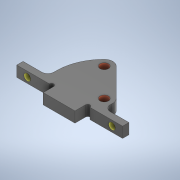
# Autodesk Inventor part: Camera_side_frame
Saved by Autodesk Inventor 2020 (Build 240168000, 168)
## iProperties
Part Number: Camera_side_frame
Material: アセタール樹脂、黒
Document SubType Name: Modeling
Designer: Masato Kubotera
Density: 1.425 g/cm^3
Appearance: 滑らか - 黒
Mass: 4.22239 g
Surface Area: 20.7437 cm^2
Volume: 2.96308 cm^3
Description: POM T5
Author: Masato Kubotera
Autodesk Inventor part; units mm, degrees
ref_plane "YZ Plane" through (0, 0, 0) normal (1, 0, 0) x (0, 1, 0)
ref_plane "XZ Plane" through (0, 0, 0) normal (0, 1, 0) x (-1, 0, 0)
ref_plane "XY Plane" through (0, 0, 0) normal (0, 0, 1) x (1, 0, 0)
derived "Head_basis.ipt"
sketch "スケッチ1" plane through (0, 0, 0) normal (0, 1, 0) x (-1, 0, 0)
  line L0 (-42.9267, 78.5217) -> (-71.5015, 49.9469) construction
  line L1 (6.295, 37.8) -> (-10.705, 37.8) construction
  line L2 (-2.205, 37.8) -> (-42.9267, 78.5217) construction
  line L3 (-2.205, 37.8) -> (-2.205, 4.9887) construction
  line L4 (-54.8845, 55.9573) -> (-58.42, 59.4928) construction
  line L5 (-58.42, 59.4928) -> (-81.0474, 36.8654) construction
  line L6 (-81.0474, 36.8654) -> (-77.5119, 33.3299) construction
  line L7 (-77.5119, 33.3299) -> (-54.8845, 55.9573) construction
  line L8 (-54.8845, 55.9573) -> (-81.0474, 36.8654) construction
  line L9 (-58.42, 59.4928) -> (-77.5119, 33.3299) construction
  line L10 (-60.2972, 54.08) -> (-70.9038, 43.4734) construction
  circle A0 centre (-60.1878, 54.1895) radius 1.6 construction
  line L11 (-56.6522, 57.725) -> (-79.2796, 35.0976) construction
  line L12 (3.8601, -2.5) -> (3.8601, 2.5) construction
  line L13 (5.295, -2.5) -> (5.295, 2.5)
  line L14 (10.8483, 2.5) -> (7.6861, 2.5) construction
  line L15 (-9.705, -2.5) -> (-9.705, 2.5)
  line L16 (5.6869, 2.5) -> (7.6861, 2.5) construction
  arc A1 (5.295, -2.5) -> (7.395, -2.5) centre (6.345, -2.5) ccw
  line L17 (9.935, -2.5) -> (11.935, -2.5) construction
  line L18 (7.395, -2.5) -> (22.795, -2.5)
  line L19 (22.795, -2.5) -> (22.795, -5.5)
  line L20 (22.795, -5.5) -> (14.045, -5.5)
  line L21 (17.795, -2.5) -> (17.795, -5.5) construction
  arc A2 (-11.805, -2.5) -> (-9.705, -2.5) centre (-10.755, -2.5) ccw
  line L22 (-11.805, -2.5) -> (-27.205, -2.5)
  line L23 (-27.205, -2.5) -> (-27.205, -5.5)
  line L24 (-22.205, -2.5) -> (-22.205, -5.5) construction
  line L25 (-18.455, -5.5) -> (-27.205, -5.5)
  circle A3 centre (-11.5577, -9.5) radius 2
  arc A4 (14.045, -5.5) -> (11.1091, -8.5601) centre (14.045, -8.4384) ccw
  line L26 (15.045, -5.5) -> (15.045, -6.9) construction
  line L27 (15.045, -6.9) -> (20.545, -6.9) construction
  line L28 (20.545, -5.5) -> (20.545, -6.9) construction
  circle A5 centre (-11.5577, -9.5) radius 4
  line L29 (22.795, -2.5) -> (22.795, 0.5)
  line L30 (-2.205, -12.0113) -> (-2.205, 4.9887) construction
  line L31 (-19.455, -5.5) -> (-19.455, -6.9) construction
  line L32 (-19.455, -6.9) -> (-24.955, -6.9) construction
  line L33 (-24.955, -5.5) -> (-24.955, -6.9) construction
  line L34 (-69.7337, 48.1791) -> (-66.1982, 44.6436) construction
  circle A6 centre (-75.7441, 38.6332) radius 1.6
  circle A7 centre (1.6555, -22.7132) radius 2
  arc A8 (4.4839, -25.5416) -> (11.1091, -8.5601) centre (-11.5577, -9.5) ccw
  line L35 (-14.3861, -12.3284) -> (-1.1729, -25.5416)
  circle A9 centre (1.6555, -22.7132) radius 4
  line L36 (4.4839, -19.8848) -> (-8.7293, -6.6716)
  line L37 (1.6555, -22.7132) -> (-11.5577, -9.5) construction
  line L38 (-49.2969, -23.1777) -> (-31.6192, -5.5) construction
  line L39 (-31.6192, -5.5) -> (-28.0837, -9.0355) construction
  line L40 (-28.0837, -9.0355) -> (-45.7614, -26.7132) construction
  line L41 (-45.7614, -26.7132) -> (-49.2969, -23.1777) construction
  line L42 (-49.2969, -23.1777) -> (-28.0837, -9.0355) construction
  line L43 (-31.6192, -5.5) -> (-45.7614, -26.7132) construction
  line L44 (-47.5291, -24.9454) -> (-29.8515, -7.2678) construction
  line L45 (-40.4581, -14.3388) -> (-36.9225, -17.8744) construction
  line L46 (-40.1045, -21.0563) -> (-33.7405, -14.6924) construction
  line L47 (-33.7405, -14.6924) -> (-37.2761, -11.1569) construction
  line L48 (-37.2761, -11.1569) -> (-43.64, -17.5208) construction
  line L49 (-43.64, -17.5208) -> (-40.1045, -21.0563) construction
  line L50 (-40.1045, -21.0563) -> (-37.2761, -11.1569) construction
  line L51 (-33.7405, -14.6924) -> (-43.64, -17.5208) construction
  circle A10 centre (-45.4078, -22.8241) radius 1.6
  line L52 (-42.2258, -16.0359) -> (-38.761, -12.5711)
  line L53 (-37.2761, -11.0861) -> (-33.6698, -14.6924)
  line L54 (-35.1548, -16.1773) -> (-38.6196, -19.6421)
  line L55 (-40.1045, -21.1271) -> (-43.7107, -17.5208)
  line L56 (-43.7107, -17.5208) -> (-33.6698, -14.6924) construction
  line L57 (-37.2761, -11.0861) -> (-40.1045, -21.1271) construction
  arc A11 (-42.2258, -16.0359) -> (-43.7107, -17.5208) centre (-42.9683, -16.7784) ccw
  arc A12 (-37.2761, -11.0861) -> (-38.761, -12.5711) centre (-38.0185, -11.8286) ccw
  circle A13 centre (-31.9728, -9.3891) radius 1.6
  line L58 (-41.8723, -19.2886) -> (-35.5083, -12.9246) construction
  arc A14 (-40.1045, -21.1271) -> (-38.6196, -19.6421) centre (-39.362, -20.3846) ccw
  arc A15 (-35.1548, -16.1773) -> (-33.6698, -14.6924) centre (-34.4123, -15.4349) ccw
  circle A16 centre (-33.205, -2.5) radius 1 construction
  line L59 (-11.5577, -5.5) -> (-31.6192, -5.5)
  line L60 (-58.42, 59.4928) -> (-54.8845, 55.9573)
  line L61 (-81.0474, 36.8654) -> (-58.42, 59.4928)
  line L62 (-45.7614, -26.7132) -> (1.6555, -26.7132)
  line L63 (-45.7614, -26.7132) -> (-49.2969, -23.1777)
  arc A17 (-15.5141, -8.9111) -> (-18.455, -5.5) centre (-18.455, -8.4733) ccw
  line L64 (-49.2969, 12.1777) -> (-45.7614, 8.6421) construction
  line L65 (-45.7614, 8.6421) -> (-63.439, -9.0355) construction
  line L66 (-49.2969, 12.1777) -> (-63.439, -9.0355) construction
  arc A18 (-59.9035, 1.6418) -> (-61.3884, 0.1569) centre (-60.646, 0.8993) ccw
  line L67 (-52.8324, 1.5004) -> (-56.2972, -1.9645)
  line L68 (-57.7822, -3.4494) -> (-61.3884, 0.1569)
  line L69 (-61.3177, 0.1569) -> (-57.7822, -3.3787) construction
  line L70 (-66.9746, -5.5) -> (-49.2969, 12.1777) construction
  line L71 (-58.1357, 3.3388) -> (-54.6002, -0.1967) construction
  arc A19 (-57.7822, -3.4494) -> (-56.2972, -1.9645) centre (-57.0397, -2.7069) ccw
  line L72 (-59.5499, -1.6109) -> (-53.186, 4.753) construction
  line L73 (-59.9035, 1.6418) -> (-56.4387, 5.1066)
  line L74 (-51.4182, 2.9853) -> (-61.3177, 0.1569) construction
  line L75 (-61.3884, 0.1569) -> (-51.3475, 2.9853) construction
  arc A20 (-52.8324, 1.5004) -> (-51.3475, 2.9853) centre (-52.09, 2.2428) ccw
  line L76 (-57.7822, -3.3787) -> (-51.4182, 2.9853) construction
  line L77 (-54.9537, 6.5208) -> (-61.3177, 0.1569) construction
  arc A21 (-54.9537, 6.5915) -> (-56.4387, 5.1066) centre (-55.6962, 5.8491) ccw
  line L78 (-57.7822, -3.3787) -> (-54.9537, 6.5208) construction
  line L79 (-51.4182, 2.9853) -> (-54.9537, 6.5208) construction
  line L80 (-54.9537, 6.5915) -> (-51.3475, 2.9853)
  circle A22 centre (-49.6504, 8.2886) radius 1.6
  line L81 (-66.9746, -5.5) -> (-45.7614, 8.6421) construction
  line L82 (-65.2068, -7.2678) -> (-47.5291, 10.4099) construction
  line L83 (-54.9537, 6.5915) -> (-57.7822, -3.4494) construction
  line L84 (-63.439, -9.0355) -> (-66.9746, -5.5) construction
  circle A23 centre (-63.0855, -5.1464) radius 1.6
  line L85 (-63.439, -9.0355) -> (-66.9746, -5.5)
  line L86 (-31.6192, -5.5) -> (-45.7614, 8.6421)
  line L87 (-49.2969, 12.1777) -> (-45.7614, 8.6421)
  line L88 (-49.2969, 12.1777) -> (-54.8845, 55.9573)
  line L89 (-63.439, -9.0355) -> (-49.2969, -23.1777)
  line L90 (-54.8845, 55.9573) -> (-77.5119, 33.3299) construction
  line L91 (-58.0382, 41.1734) -> (-54.6915, 14.9518)
  line L92 (-55.2612, 13.2844) -> (-62.4919, 6.0537)
  line L93 (-65.8041, 6.8374) -> (-73.177, 29.0328)
  line L94 (-72.6932, 31.0775) -> (-61.4363, 42.3344)
  arc A24 (-58.0382, 41.1734) -> (-61.4363, 42.3344) centre (-60.0221, 40.9202) ccw
  arc A25 (-72.6932, 31.0775) -> (-73.177, 29.0328) centre (-71.2789, 29.6633) ccw
  arc A26 (-65.8041, 6.8374) -> (-62.4919, 6.0537) centre (-63.9061, 7.4679) ccw
  arc A27 (-55.2612, 13.2844) -> (-54.6915, 14.9518) centre (-56.6754, 14.6986) ccw
  line L95 (-15.4866, -18.299) -> (-21.4671, -12.3185)
  line L96 (-24.2956, -12.3185) -> (-30.2761, -18.299)
  line L97 (-28.8619, -21.7132) -> (-16.9008, -21.7132)
  arc A28 (-16.9008, -21.7132) -> (-15.4866, -18.299) centre (-16.9008, -19.7132) ccw
  arc A29 (-21.4671, -12.3185) -> (-24.2956, -12.3185) centre (-22.8813, -13.7327) ccw
  arc A30 (-30.2761, -18.299) -> (-28.8619, -21.7132) centre (-28.8619, -19.7132) ccw
  line L98 (-40.1045, -4.0858) -> (-44.3471, 0.1569)
  line L99 (-47.1756, 0.1569) -> (-54.9537, -7.6213)
  line L100 (-54.9537, -10.4497) -> (-50.7111, -14.6924)
  line L101 (-47.8827, -14.6924) -> (-40.1045, -6.9142)
  arc A31 (-40.1045, -6.9142) -> (-40.1045, -4.0858) centre (-41.5187, -5.5) ccw
  arc A32 (-44.3471, 0.1569) -> (-47.1756, 0.1569) centre (-45.7614, -1.2574) ccw
  arc A33 (-54.9537, -7.6213) -> (-54.9537, -10.4497) centre (-53.5395, -9.0355) ccw
  arc A34 (-50.7111, -14.6924) -> (-47.8827, -14.6924) centre (-49.2969, -13.2782) ccw
  circle A35 centre (-11.5577, -9.5) radius 1.6
  circle A36 centre (1.6555, -22.7132) radius 1.6
  line L102 (-61.9555, 48.8862) -> (-70.4408, 40.4009) construction
  line L103 (-70.4408, 40.4009) -> (-72.2086, 42.1687) construction
  line L104 (-72.2086, 42.1687) -> (-63.7233, 50.654) construction
  line L105 (-63.7233, 50.654) -> (-61.9555, 48.8862) construction
  line L106 (-61.9555, 48.8862) -> (-72.2086, 42.1687) construction
  line L107 (-70.4408, 40.4009) -> (-63.7233, 50.654) construction
  line L108 (-62.8394, 49.7701) -> (-71.3247, 41.2848) construction
  line L109 (-61.8848, 48.8862) -> (-63.7233, 50.7247)
  line L110 (-63.7233, 50.7247) -> (-72.2793, 42.1687)
  line L111 (-72.2793, 42.1687) -> (-70.4408, 40.3302)
  line L112 (-70.4408, 40.3302) -> (-61.8848, 48.8862)
  line L113 (-61.8848, 48.8862) -> (-72.2793, 42.1687) construction
  line L114 (-63.7233, 50.7247) -> (-70.4408, 40.3302) construction
  arc A37 (-63.3697, 47.4013) -> (-61.8848, 48.8862) centre (-62.6273, 48.1437) ccw
  arc A38 (-62.6733, 49.6747) -> (-64.7733, 49.6747) centre (-63.7233, 49.6747) ccw
  arc A39 (-70.4408, 40.3302) -> (-68.9559, 41.8151) centre (-69.6983, 41.0727) ccw
  arc A40 (-71.2293, 43.2187) -> (-71.2293, 41.1187) centre (-71.2293, 42.1687) ccw
  line L115 (-9.705, 2.5) -> (5.295, 2.5)
  line L116 (-16.595, 2.5) -> (12.185, 2.5)
  line L117 (-2.205, 2.5) -> (-60.5767, 60.8717) construction
  line L118 (-66.9746, -5.5) -> (-81.0474, 36.8654)
  line L119 (-22.205, -2.5) -> (17.795, -2.5)
  line L120 (-71.5015, 49.9469) -> (-60.5767, 60.8717) construction
  line L121 (-32.205, 2.4749) -> (-32.205, 30.3)
  point P0 (-67.9659, 46.4113)
  point P1 (-14.345, -2.5)
  point P2 (-9.705, -2.5)
  point P3 (-14.305, -2.5)
  point P4 (9.895, -2.5)
  point P5 (-38.6903, -16.1066)
  point P6 (-38.6903, -16.1066)
  point P7 (-56.368, 1.5711)
  point P8 (-56.368, 1.5711)
  point P9 (-54.5673, 13.9784)
  point P10 (-67.0821, 45.5274)
  point P11 (-67.0821, 45.5274)
  dimension "d5" = 5
  measures "d5" distance of L21.start L18.end
extrude "押し出し1" add sketch "スケッチ1" along normal blind 5 contours L119 L15 L115 L13 | A1 L18 L19 L20 A4 A8 A9 L36 A5 L59 L25 L23 L22 A2 L119 | L59 A5 A17 | A9 | A5 | L36 A9 L35 A5
sketch "スケッチ2" plane through (-22.795, 0, -2.5) normal (0, 0, 1) x (1, 0, 0)
  line L0 (5, 0) -> (5, 5) construction
  line L1 (50, 0) -> (50, 5) projected
  line L2 (0, 5) -> (50, 5)
  line L3 (0, 0) -> (15.4, 0) projected
  line L4 (34.6, 0) -> (50, 0) projected
  line L5 (0, 0) -> (50, 0)
  line L6 (25, 5) -> (25, 0)
  line L7 (0, 5) -> (15.4, 5) projected
  point P0 (5, 2.5)
  point P1 (45, 2.5)
  dimension "d13" = 5
  constraints: 8 end point, 3 midpoint, 2 horizontal, 2 point on line, 1 perpendicular, 1 symmetric about line
  measures "d13" distance of L2.start L0.end
hole "穴1" at (-17.795, 2.5, -2.5) at (22.205, 2.5, -2.5) direction (0, 0, -1) diameter 3.2 end through all
